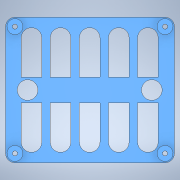
# Autodesk Inventor part: Pi_mount
Saved by Autodesk Inventor 2022 (Build 260153000, 153)
## iProperties
Created: 2023-01-21
Part Number: Pi_mount
Material: Generic
Document SubType Name: Modeling
Designer: Harmonic Ash
Density: 1 g/cm^3
Appearance: Default
Author: Harmonic Ash
Autodesk Inventor part; units mm, degrees
ref_plane "YZ Plane" through (0, 0, 0) normal (1, 0, 0) x (0, 1, 0)
sketch "Sketch1" plane through (0, 0, 0) normal (0, 1, 0) x (-1, 0, 0)
  circle A0 centre (0, 0) radius 3.1
  circle A1 centre (49, 0) radius 3.1
  circle A2 centre (49, -58) radius 3.1
  circle A3 centre (0, -58) radius 3.1
  dimension "d4" = 6.2
  dimension "d5" = 6.2
  dimension "d6" = 6.2
  dimension "d7" = 6.2
  dimension "d12" = 58
  dimension "d13" = 58
  dimension "d14" = 49
  dimension "d15" = 49
  constraints: 4 centre point
  measures "d4" diameter of A0
  measures "d5" diameter of A1
  measures "d6" diameter of A2
  measures "d7" diameter of A3
  measures "d12" distance of A3.centre point (0, 0)
  measures "d13" distance of A2.centre A1.centre
  measures "d14" distance of point (0, 0) A1.centre
  measures "d15" distance of A3.centre A2.centre
extrude "Extrusion1" add sketch "Sketch1" along normal blind 2
sketch "Sketch3" plane through (0, 2, 0) normal (0, 1, 0) x (1, 0, 0)
  circle A0 centre (0, 0) radius 3.1 projected
  circle A1 centre (0, 0) radius 3.625
  circle A2 centre (0, 58) radius 3.1 projected
  circle A3 centre (0, 58) radius 3.625
  circle A4 centre (-49, 58) radius 3.1 projected
  circle A5 centre (-49, 58) radius 3.625
  circle A6 centre (-49, 0) radius 3.1 projected
  circle A7 centre (-49, 0) radius 3.625
  line L0 (-52.625, 0) -> (-52.625, 58)
  line L1 (-49, 61.625) -> (0, 61.625)
  line L2 (3.625, 58) -> (3.625, 0)
  line L3 (0, -3.625) -> (-49, -3.625)
  dimension "d18" = 7.25
  dimension "d19" = 7.25
  dimension "d20" = 7.25
  dimension "d21" = 7.25
  constraints: 8 end point, 8 point on circle, 6 tangent, 4 centre point, 4 coincident, 1 vertical
  measures "d18" diameter of A1
  measures "d19" diameter of A3
  measures "d20" diameter of A5
  measures "d21" diameter of A7
extrude "Extrusion2" add sketch "Sketch3" along normal blind 2 contours A0 | A1 | A1 L3 A7 L0 A5 L1 A3 L2 | A3 | A7 | A5 | A2 | A4 | A6
sketch "Sketch5" plane through (0, 2, 0) normal (0, -1, 0) x (1, 0, 0)
  circle A0 centre (-4.375, -6.375) radius 4
  circle A1 centre (-44.625, -6.375) radius 4
  line L0 (3.625, 0) -> (3.625, -58) projected
  line L1 (-52.625, -58) -> (-52.625, 0) projected
  line L2 (-49, 3.625) -> (0, 3.625) projected
  line L3 (-4.375, -2.375) -> (-44.625, -2.375)
  line L4 (-4.375, -10.375) -> (-44.625, -10.375)
  circle A2 centre (-4.375, -17.625) radius 4
  line L5 (-4.375, -13.625) -> (-44.625, -13.625)
  line L6 (-4.375, -21.625) -> (-44.625, -21.625)
  circle A3 centre (-44.625, -17.625) radius 4
  circle A4 centre (-4.375, -28.875) radius 4
  line L7 (-4.375, -24.875) -> (-44.625, -24.875)
  line L8 (-4.375, -32.875) -> (-44.625, -32.875)
  circle A5 centre (-44.625, -28.875) radius 4
  circle A6 centre (-4.375, -40.125) radius 4
  line L9 (-4.375, -36.125) -> (-44.625, -36.125)
  line L10 (-4.375, -44.125) -> (-44.625, -44.125)
  circle A7 centre (-44.625, -40.125) radius 4
  circle A8 centre (-4.375, -51.375) radius 4
  line L11 (-4.375, -47.375) -> (-44.625, -47.375)
  line L12 (-4.375, -55.375) -> (-44.625, -55.375)
  circle A9 centre (-44.625, -51.375) radius 4
  point P0 (0, 0)
  dimension "d27" = 8
  dimension "d28" = 8
  dimension "d29" = 8
  dimension "d30" = 8
  dimension "d31" = 10
  dimension "d32" = 10
  dimension "d35" = 11.25
  constraints: 20 end point, 20 point on circle, 10 centre point, 2 tangent, 1 horizontal, 1 vertical, 40 other
  measures "d27" diameter of A0
  measures "d28" diameter of A1
  measures "d29" distance from line of L0 A0.centre
  measures "d30" distance from line of L1 A1.centre
  measures "d31" distance from line of L2 A1.centre
  measures "d32" distance from line of L2 A0.centre
  measures "d35" distance of A0.centre A2.centre
extrude "Extrusion3" cut sketch "Sketch5" against normal blind 2
sketch "Sketch6" plane through (0, 0, 0) normal (0, -1, 0) x (1, 0, 0)
  circle A0 centre (0, 0) radius 3.1 projected
  circle A1 centre (-49, -58) radius 3.1 projected
  line L0 (0, 0) -> (-49, 0)
  line L1 (-49, 0) -> (-49, -58)
  line L2 (-49, -58) -> (0, -58)
  line L3 (0, -58) -> (0, 0)
  constraints: 8 end point, 2 parallel, 1 horizontal, 1 perpendicular
hole "Hole1" at (0, 0, -58) at (0, 0, 0) at (-49, 0, 0) at (-49, 0, -58) direction (0, 1, 0) diameter 2 end through all
sketch "Sketch7" plane through (0, 4, 0) normal (0, 1, 0) x (1, 0, 0)
  circle A0 centre (-24.5, 52.875) radius 4
  circle A1 centre (-24.5, 4.875) radius 4
  line L0 (-49, -3.625) -> (0, -3.625) projected
  point P0 (0, 0)
  dimension "d49" = 8
  dimension "d50" = 8
  dimension "d51" = 48
  dimension "d52" = 8.5
  constraints: 2 centre point
  measures "d49" diameter of A0
  measures "d50" diameter of A1
  measures "d51" distance of A1.centre A0.centre
  measures "d52" distance from line of L0 A1.centre
ref_plane "Work Plane2" through (0, 4, 0) normal (0, -1, 0) x (1, 0, 0)
sketch "Sketch8" plane through (0, 4, 0) normal (0, -1, 0) x (1, 0, 0)
  line L0 (-29.5, -61.5) -> (-19.5, -61.5)
  line L1 (-19.5, -61.5) -> (-19.5, 3.5)
  line L2 (-19.5, 3.5) -> (-29.5, 3.5)
  line L3 (-29.5, 3.5) -> (-29.5, -61.5)
  arc A0 (-27.6225, -2.5) -> (-21.3775, -2.5) centre (-24.5, -5) ccw projected
  point P0 (0, 0)
  dimension "d55" = 10
  dimension "d56" = 5
  constraints: 8 end point, 2 parallel, 1 horizontal, 1 perpendicular
  measures "d55" distance of L2.end L1.end
  measures "d56" distance from line of A0.centre L1
extrude "Extrusion5" add sketch "Sketch8" along normal up to surface (2 mm away)
ref_plane "Work Plane1" through (-24.5, 7, -5) normal (0, 1, 0) x (1, 0, 0)
extrude "Extrusion6" cut sketch "Sketch7" against normal blind 10
equation "\"d18\" = d19"
equation "\"d20\" = d19"
equation "\"d21\" = d19"
body "Solid1"
